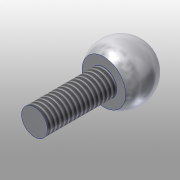
# Autodesk Inventor part: 500-113
Saved by Autodesk Inventor 2016 (Build 200138000, 138)
## iProperties
Created: 2015-04-18
Part Number: 500-113
Material: Aluminum 6061
Document SubType Name: Modeling
Designer: Station9
Density: 2.7 g/cm^3
Appearance: Aluminum - Flat
Mass: 0.459187 g
Surface Area: 2.14878 cm^2
Volume: 0.170069 cm^3
Author: Station9
Autodesk Inventor part; units mm, degrees
ref_plane "YZ Plane" through (0, 0, 0) normal (1, 0, 0) x (0, 1, 0)
ref_plane "XZ Plane" through (0, 0, 0) normal (0, 1, 0) x (-1, 0, 0)
ref_plane "XY Plane" through (0, 0, 0) normal (0, 0, 1) x (1, 0, 0)
sketch "Sketch1" plane through (0, 0, 0) normal (0, 1, 0) x (-1, 0, 0)
  circle A0 centre (0, 0) radius 3.2
  line L0 (3.2, 0) -> (-3.2, 0)
  dimension "d0" = 6.4
  constraints: 2 end point, 2 point on circle, 1 centre point, 1 coincident, 1 horizontal
  measures "d0" diameter of A0
revolve "Revolution1" add sketch "Sketch1" angle 360 about axis through (-3.2, 0, 0) along (1, 0, 0) picked at (1.0667, -1.9947) contours A0 L0
sketch "Sketch2" plane through (0, 0, 0) normal (1, 0, 0) x (0, 1, 0)
  line L0 (-1.9733, 5.6826) -> (-7.2021, 5.6826)
  line L1 (-7.2021, 5.6826) -> (-7.2021, -6.4165)
  line L2 (-7.2021, -6.4165) -> (-1.9733, -6.4165)
  line L3 (-1.9733, -6.4165) -> (-1.9733, 5.6826)
  line L4 (5.3731, 6.6744) -> (2.8267, 6.6744)
  line L5 (2.8267, 6.6744) -> (2.8267, -5.9008)
  line L6 (2.8267, -5.9008) -> (5.3731, -5.9008)
  line L7 (5.3731, -5.9008) -> (5.3731, 6.6744)
  circle A0 centre (0, 0) radius 3.2 projected
  point P0 (2.8267, -1.5)
  point P1 (2.8267, 1.5)
  dimension "d2" = 4.8
  dimension "d8" = 3
  constraints: 16 end point, 4 parallel, 2 horizontal, 2 perpendicular, 2 point on circle, 2 point on line
  measures "d2" distance between parallel lines of L3 L5
  measures "d8" distance of A0.end A0.start
extrude "Extrusion1" cut sketch "Sketch2" along normal mid plane 10 contours L3 A0 L2 L1 L0 | L3 A0 | A0 L5 | L5 L4 L7 L6 A0
sketch "Sketch3" plane through (0, -1.9733, 0) normal (0, -1, 0) x (1, 0, 0)
  circle A0 centre (0, 0) radius 2.5191 projected
  circle A1 centre (0, 0) radius 1.5
  dimension "d5" = 3
  constraints: 1 centre point, 1 coincident
  measures "d5" diameter of A1
extrude "Extrusion2" add sketch "Sketch3" along normal blind 8 contours A1
thread "Thread1" size "M3x0.5" class "6g" standard "ANSI Metric M Profile" full length
sketch "Sketch4" plane through (0, 2.8267, 0) normal (0, 1, 0) x (1, 0, 0)
  line L0 (-1.3899, 0) -> (-0.7247, 1.1522)
  line L1 (-0.7247, 1.1522) -> (0.6057, 1.1522)
  line L2 (0.6057, 1.1522) -> (1.2709, 0)
  line L3 (1.2709, 0) -> (0.6057, -1.1522)
  line L4 (0.6057, -1.1522) -> (-0.7247, -1.1522)
  line L5 (-0.7247, -1.1522) -> (-1.3899, 0)
  point P0 (-0.0595, 0)
  constraints: 12 end point, 13 other
extrude "Extrusion3" cut sketch "Sketch4" against normal blind 2
body "Solid1"
